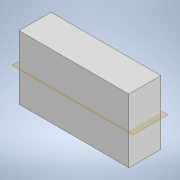
# Autodesk Inventor part: Receiver
Saved by Autodesk Inventor 2021 (Build 250183000, 183)
## iProperties
Created: 2020-11-24
Part Number: Receiver
Material: Generic
Document SubType Name: Modeling
Designer: Kanenas
Mass: 9.6 g
Surface Area: 38.5 cm^2
Volume: 13.4375 cm^3
Density: 0.714419 g/cm^3
Appearance: Default
Author: Kanenas
Autodesk Inventor part; units mm, degrees
ref_plane "YZ Plane" through (0, 0, 0) normal (1, 0, 0) x (0, 1, 0)
ref_plane "XY Plane" through (0, 0, 0) normal (0, 0, 1) x (1, 0, 0)
sketch "Sketch1" plane through (0, 0, 0) normal (0, 0, 1) x (1, 0, 0)
  line L0 (-21.5, 12.5) -> (21.5, 12.5)
  line L1 (21.5, 12.5) -> (21.5, -12.5)
  line L2 (21.5, -12.5) -> (-21.5, -12.5)
  line L3 (-21.5, -12.5) -> (-21.5, 12.5)
  line L4 (-21.5, 12.5) -> (21.5, -12.5) construction
  line L5 (21.5, 12.5) -> (-21.5, -12.5) construction
  point P0 (0, 0)
  dimension "d0" = 43
  dimension "d1" = 25
  constraints: 12 end point, 2 midpoint, 2 parallel, 1 horizontal, 1 perpendicular
  measures "d0" distance of L0.start L0.end
  measures "d1" distance of L0.end L1.end
extrude "Extrusion1" add sketch "Sketch1" along normal blind 12.5
body "Solid1"
